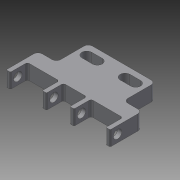
# Autodesk Inventor part: tubing_connection_holder
Saved by Autodesk Inventor 2015 (Build 190159000, 159)
## iProperties
Created: 2017-04-05
Part Number: tubing_connection_holder
Material: Generic
Document SubType Name: Modeling
Designer: Guy
Density: 1 g/cm^3
Appearance: Default
Author: Guy
Autodesk Inventor part; units mm, degrees
ref_plane "YZ Plane" through (0, 0, 0) normal (1, 0, 0) x (0, 1, 0)
ref_plane "XZ Plane" through (0, 0, 0) normal (0, 1, 0) x (-1, 0, 0)
ref_plane "XY Plane" through (0, 0, 0) normal (0, 0, 1) x (1, 0, 0)
sketch "Sketch1" plane through (0, 0, 0) normal (0, 0, 1) x (1, 0, 0)
  line L0 (0, 0) -> (49, 0)
  line L1 (49, 0) -> (49, 30)
  line L2 (49, 30) -> (0, 30)
  line L3 (0, 30) -> (0, 0)
  dimension "d0" = 30
  dimension "d1" = 49
  constraints: 8 end point, 2 parallel, 1 horizontal, 1 perpendicular
  measures "d0" distance of L2.end L0.start
  measures "d1" distance of L1.end L2.end
extrude "Extrusion1" add sketch "Sketch1" along normal blind 7
sketch "Sketch2" plane through (0, 0, 7) normal (0, 0, 1) x (1, 0, 0)
  arc A0 (12.975, 27.3) -> (12.975, 22.7) centre (12.975, 25) ccw
  arc A1 (17.975, 22.7) -> (17.975, 27.3) centre (17.975, 25) ccw
  arc A2 (31.025, 27.3) -> (31.025, 22.7) centre (31.025, 25) ccw
  arc A3 (36.025, 22.7) -> (36.025, 27.3) centre (36.025, 25) ccw
  line L0 (12.975, 27.3) -> (17.975, 27.3)
  line L1 (12.975, 22.7) -> (17.975, 22.7)
  line L2 (31.025, 27.3) -> (36.025, 27.3)
  line L3 (31.025, 22.7) -> (36.025, 22.7)
  line L4 (49, 30) -> (0, 30) projected
  line L5 (0, 30) -> (0, 0) projected
  dimension "d4" = 4.6
  dimension "d5" = 4.6
  dimension "d6" = 4.6
  dimension "d8" = 5
  dimension "d9" = 5
  dimension "d10" = 13.05
  dimension "d11" = 5
  dimension "d12" = 12.975
  dimension "d13" = 49
  dimension "d17" = 2.3
  constraints: 8 end point, 8 point on circle, 6 tangent, 4 centre point, 2 horizontal, 2 parallel, 1 collinear
  measures "d4" diameter of A0
  measures "d5" diameter of A1
  measures "d6" diameter of A2
  measures "d8" distance of A1.centre A0.centre
  measures "d9" distance of A3.centre A2.centre
  measures "d10" distance of A2.centre A1.centre
  measures "d11" distance from line of A0.centre L4
  measures "d12" distance from line of L5 A0.centre
  measures "d13" distance of L4.start L4.end
  measures "d17" radius of A3
extrude "Extrusion2" cut sketch "Sketch2" against normal up to next
sketch "Sketch3" plane through (0, 0, 7) normal (0, 0, 1) x (1, 0, 0)
  arc A0 (12.975, 27.3) -> (12.975, 22.7) centre (12.975, 25) ccw projected
  line L0 (12.975, 27.3) -> (17.975, 27.3) projected
  arc A1 (17.975, 22.7) -> (17.975, 27.3) centre (17.975, 25) ccw projected
  line L1 (17.975, 22.7) -> (12.975, 22.7) projected
  arc A2 (31.025, 27.3) -> (31.025, 22.7) centre (31.025, 25) ccw projected
  line L2 (31.025, 27.3) -> (36.025, 27.3) projected
  arc A3 (36.025, 22.7) -> (36.025, 27.3) centre (36.025, 25) ccw projected
  line L3 (36.025, 22.7) -> (31.025, 22.7) projected
  line L4 (0, 0) -> (49, 0) projected
  line L5 (49, 0) -> (49, 30) projected
  line L6 (49, 30) -> (0, 30) projected
  line L7 (0, 30) -> (0, 0) projected
  line L8 (2, 8) -> (17, 8)
  line L9 (17, 8) -> (17, 0)
  line L10 (17, 0) -> (2, 0)
  line L11 (2, 0) -> (2, 8)
  line L12 (32, 8) -> (47, 8)
  line L13 (47, 8) -> (47, 0)
  line L14 (47, 0) -> (32, 0)
  line L15 (32, 0) -> (32, 8)
  line L16 (0, 0) -> (49, 0) projected
  line L17 (19, 0) -> (30, 0)
  line L18 (30, 0) -> (30, 8)
  line L19 (30, 8) -> (19, 8)
  line L20 (19, 8) -> (19, 0)
  dimension "d18" = 8
  dimension "d19" = 15
  dimension "d20" = 15
  dimension "d21" = 15
  dimension "d22" = 2
  dimension "d23" = 49
  dimension "d35" = 2
  dimension "d36" = 2
  constraints: 24 end point, 6 parallel, 4 point on line, 3 horizontal, 3 perpendicular, 1 collinear
  measures "d18" distance of L10.end L8.start
  measures "d19" distance of L8.start L8.end
  measures "d20" distance of L12.start L12.end
  measures "d21" distance between parallel lines of L9 L15
  measures "d22" distance between parallel lines of L5 L13
  measures "d23" distance of L5.end L6.end
  measures "d35" distance between parallel lines of L18 L15
  measures "d36" distance between parallel lines of L9 L20
sketch "Sketch4" plane through (0, 0, 7) normal (0, 0, 1) x (1, 0, 0)
  arc A0 (12.975, 27.3) -> (12.975, 22.7) centre (12.975, 25) ccw projected
  line L0 (12.975, 27.3) -> (17.975, 27.3) projected
  arc A1 (17.975, 22.7) -> (17.975, 27.3) centre (17.975, 25) ccw projected
  line L1 (17.975, 22.7) -> (12.975, 22.7) projected
  arc A2 (31.025, 27.3) -> (31.025, 22.7) centre (31.025, 25) ccw projected
  line L2 (31.025, 27.3) -> (36.025, 27.3) projected
  arc A3 (36.025, 22.7) -> (36.025, 27.3) centre (36.025, 25) ccw projected
  line L3 (36.025, 22.7) -> (31.025, 22.7) projected
  line L4 (0, 0) -> (49, 0) projected
  line L5 (49, 0) -> (49, 30) projected
  line L6 (49, 30) -> (0, 30) projected
  line L7 (0, 30) -> (0, 0) projected
  line L8 (0, 30) -> (8.675, 30)
  line L9 (8.675, 30) -> (8.675, 15)
  line L10 (8.675, 15) -> (0, 15)
  line L11 (0, 15) -> (0, 30)
  line L12 (49, 30) -> (40.325, 30)
  line L13 (40.325, 30) -> (40.325, 15)
  line L14 (40.325, 15) -> (49, 15)
  line L15 (49, 15) -> (49, 30)
  dimension "d26" = 8.675
  dimension "d27" = 8.675
  dimension "d28" = 30
  dimension "d29" = 15
  dimension "d31" = 2.3
  dimension "d32" = 12.975
  constraints: 16 end point, 4 parallel, 2 horizontal, 2 perpendicular, 1 collinear
  measures "d26" distance between parallel lines of L11 L9
  measures "d27" distance between parallel lines of L5 L13
  measures "d28" distance of L4.end L5.end
  measures "d29" distance between parallel lines of L4 L14
  measures "d31" radius of A3
  measures "d32" distance from line of L5 A3.centre
extrude "Extrusion3" cut sketch "Sketch3" against normal up to next contours L11 L8 L9 L4 | L20 L19 L18 L4 | L4 L15 L12 L13
extrude "Extrusion4" cut sketch "Sketch4" against normal up to next contours L7 L6 L9 L10 | L14 L13 L6 L5
sketch "Sketch5" plane through (49, 0, 7) normal (1, 0, 0) x (0, 0, -1)
  circle A0 centre (3.5, 3.5) radius 2
  line L0 (0, 0) -> (0, 15) projected
  line L1 (7, 0) -> (0, 0) projected
  dimension "d37" = 4
  dimension "d38" = 3.5
  dimension "d39" = 3.5
  dimension "d40" = 7
  constraints: 1 centre point
  measures "d37" diameter of A0
  measures "d38" distance from line of A0.centre L0
  measures "d39" distance from line of A0.centre L1
  measures "d40" distance of L1.start L0.start
extrude "Extrusion5" cut sketch "Sketch5" against normal through all
fillet "Fillet1" radius 1 6 edges at (2, 8, 3.5) (17, 8, 3.5) (19, 8, 3.5) (30, 8, 3.5) (32, 8, 3.5) (47, 8, 3.5)
fillet "Fillet2" radius 2 6 edges at (40.325, 15, 3.5) (8.675, 15, 3.5) (8.675, 30, 3.5) (40.325, 30, 3.5) (49, 15, 3.5) (0, 15, 3.5)
fillet "Fillet3" radius 0.5 8 edges at (0, 0, 3.5) (2, 0, 3.5) (17, 0, 3.5) (19, 0, 3.5) (30, 0, 3.5) (32, 0, 3.5) (47, 0, 3.5) (49, 0, 3.5)
equation "\"d5\" = d4"
equation "\"d6\" = d4"
equation "\"d12\" = -0.5 * d8 - 0.5 * d9 + 0.5 * d13 - 0.5 * d10"
equation "\"d17\" = 0.5 * d6"
equation "\"d22\" = -0.5 * d20 - 0.5 * d19 + 0.5 * d23 - 0.5 * d21"
equation "\"d35\" = d22"
equation "\"d36\" = d35"
equation "\"d26\" = d27"
equation "\"d38\" = 0.5 * d40"
equation "\"d39\" = d38"
body "Solid1"
